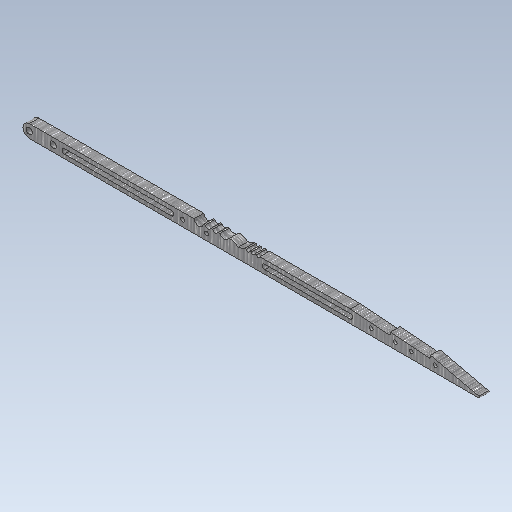
# Autodesk Inventor part: ロッド
Saved by Autodesk Inventor 2020 (Build 240168000, 168)
## iProperties
Created: 2019-12-03
Part Number: ロッド
Material: アルミニウム 7075
Document SubType Name: Modeling
Designer: tanjihayato
Density: 2.81 g/cm^3
Appearance: サテン - ブラシ仕上げ 重厚
Mass: 28.905 g
Surface Area: 93.2256 cm^2
Volume: 10.2865 cm^3
Author: tanjihayato
Autodesk Inventor part; units mm, degrees
ref_plane "YZ Plane" through (0, 0, 0) normal (1, 0, 0) x (0, 1, 0)
ref_plane "XZ Plane" through (0, 0, 0) normal (0, 1, 0) x (-1, 0, 0)
ref_plane "XY Plane" through (0, 0, 0) normal (0, 0, 1) x (1, 0, 0)
sketch "スケッチ1" plane through (0, 0, 0) normal (0, 0, 1) x (1, 0, 0)
  circle A0 centre (0, 0) radius 2
  circle A1 centre (15, 0) radius 2
  arc A2 (-0.2273, 4.9948) -> (-2.9263, -4.0542) centre (0, 0) ccw
  circle A3 centre (55, 0) radius 1.5
  circle A4 centre (55, 0) radius 4.025
  arc A5 (57.9262, 6.3865) -> (54.6807, 7.0177) centre (55, 0) ccw
  arc A6 (46.6204, -10.301) -> (48.0377, -5.2999) centre (45.4517, -7.2684) ccw
  line L0 (80, -19) -> (95, -19)
  circle A7 centre (95, -15) radius 2
  circle A8 centre (80, -15) radius 2
  arc A9 (95, -19) -> (96.6662, -11.3635) centre (95, -15) ccw
  circle A10 centre (80, -15) radius 4 construction
  line L1 (48.2385, -19) -> (80, -19)
  line L2 (57.9262, 6.3865) -> (96.6662, -11.3635)
  arc A11 (46.3293, 1.1755) -> (48.0377, -5.2999) centre (55, 0) ccw
  arc A12 (62.367, -1.4063) -> (54.6591, 7.4922) centre (55, 0) ccw
  line L3 (-0.2273, 4.9948) -> (54.6591, 7.4922)
  circle A13 centre (13, -10) radius 1.5
  arc A14 (10.3663, -13.6488) -> (12.3637, -14.4548) centre (13, -10) ccw
  line L4 (-2.9263, -4.0542) -> (10.3663, -13.6488)
  arc A15 (54.3637, -20.4538) -> (59.4202, -16.8428) centre (55, -15.999) ccw
  line L5 (12.3637, -14.4548) -> (54.3637, -20.4538)
  line L6 (59.4202, -16.8428) -> (62.367, -1.4063)
  circle A16 centre (66.7169, -2.5911) radius 1.5
  circle A17 centre (66.7169, -2.5911) radius 4.5 construction
  circle A18 centre (48.2385, -14.5) radius 1.5
  arc A19 (46.6204, -10.301) -> (48.2385, -19) centre (48.2385, -14.5) ccw
  arc A20 (80, -11) -> (80, -19) centre (80, -15) ccw
  line L7 (355.4948, -11) -> (390, -19)
  line L8 (390, -19) -> (80, -19)
  circle A21 centre (358.4948, -15) radius 1.25
  circle A22 centre (343.4948, -15) radius 1.25
  circle A23 centre (333.4948, -15) radius 1.25
  circle A24 centre (318.4948, -15) radius 1.25
  line L9 (80, -11) -> (207.8755, -11)
  line L10 (355.4948, -11) -> (248.9511, -11)
  arc A25 (213.7823, -10) -> (213.8378, -11) centre (210.8567, -10.6639) ccw
  line L11 (213.7823, -10) -> (214.7761, -9.8894)
  line L12 (213.8378, -11) -> (214.8378, -11)
  line L13 (219.357, -11) -> (218.357, -11)
  line L14 (218.2737, -9.5) -> (219.2676, -9.3894)
  line L15 (222.8762, -11) -> (223.8762, -11)
  line L16 (222.7652, -9) -> (223.7591, -8.8894)
  arc A26 (214.8378, -11) -> (218.357, -11) centre (216.5974, -10.3453) ccw
  arc A27 (218.2737, -9.5) -> (214.7761, -9.8894) centre (216.5974, -10.3453) ccw
  arc A28 (219.357, -11) -> (222.8762, -11) centre (221.1166, -10.0946) ccw
  arc A29 (222.7652, -9) -> (219.2676, -9.3894) centre (221.1166, -10.0946) ccw
  line L17 (210.8567, -10.6639) -> (233.0155, -9.4343) construction
  arc A30 (223.8762, -11) -> (229.892, -10.6107) centre (226.7628, -8.9308) ccw
  arc A31 (226.8407, -8.7739) -> (223.7591, -8.8894) centre (225.3075, -9.0352) ccw
  arc A32 (226.8407, -8.7739) -> (230.4998, -7.0068) centre (226.5478, -3.4953) ccw
  arc A33 (233.6316, -8.397) -> (230.4998, -7.0068) centre (231.2455, -9.5496) ccw
  arc A34 (235.4619, -12.6053) -> (229.892, -10.6107) centre (230.3136, -18.2076) ccw
  arc A35 (235.4619, -12.6053) -> (239.6511, -11) centre (234.0497, -2.6513) ccw
  arc A36 (259.6965, 4.4867) -> (265.8152, 14.9495) centre (248.2498, 18.2013) ccw
  arc A37 (220.191, -4.195) -> (265.8152, 14.9495) centre (219.3797, 61.6752) ccw
  line L18 (220.191, -4.195) -> (207.615, -4.3499)
  arc A38 (196.7777, -11) -> (207.615, -4.3499) centre (196.7777, 1.1554) ccw
  line L19 (222.8762, -11) -> (240.076, -10.0456) construction
  line L20 (222.7652, -9) -> (239.478, -8.0726) construction
  line L21 (239.6511, -11) -> (240.6511, -11)
  arc A39 (240.6511, -11) -> (242.7511, -11) centre (241.7011, -11) ccw
  line L22 (242.7511, -11) -> (243.7511, -11)
  arc A40 (243.7511, -11) -> (245.8511, -11) centre (244.8011, -11) ccw
  line L23 (245.8511, -11) -> (246.8511, -11)
  arc A41 (246.8511, -11) -> (248.9511, -11) centre (247.9011, -11) ccw
  arc A42 (240.735, -6.337) -> (238.7449, -7.0075) centre (239.7428, -6.6807) ccw
  arc A43 (243.5362, -5.2633) -> (241.5809, -6.0291) centre (242.5618, -5.6544) ccw
  arc A44 (246.2823, -4.0554) -> (244.3663, -4.9148) centre (245.3279, -4.4932) ccw
  arc A45 (248.9668, -2.7162) -> (247.0946, -3.6672) centre (248.0347, -3.1996) ccw
  arc A46 (233.6316, -8.397) -> (238.7449, -7.0075) centre (219.9279, 52.1342) ccw
  arc A47 (240.735, -6.337) -> (241.5809, -6.0291) centre (219.9279, 52.1342) ccw
  arc A48 (243.5362, -5.2633) -> (244.3663, -4.9148) centre (219.9279, 52.1342) ccw
  arc A49 (246.2823, -4.0554) -> (247.0946, -3.6672) centre (219.9279, 52.1342) ccw
  arc A50 (248.9668, -2.7162) -> (259.6965, 4.4867) centre (219.9279, 52.1342) ccw
  line L24 (196.7777, -11) -> (196.7777, -15)
  circle A51 centre (200.7777, -15) radius 1.25
  circle A52 centre (215.7777, -15) radius 1.25
  arc A53 (196.7777, -15) -> (200.7777, -19) centre (200.7777, -15) ccw
  arc A54 (215.7777, -19) -> (217.9536, -11.6436) centre (215.7777, -15) ccw
  circle A55 centre (200.7777, -15) radius 1.5
  circle A56 centre (215.7777, -15) radius 1.5
  line L25 (200.7777, -19) -> (215.7777, -19)
  circle A57 centre (45.4517, -7.2684) radius 1.5
  arc A58 (46.3293, 1.1755) -> (44.1782, 4.6812) centre (43.1088, 1.6121) ccw
  line L26 (54.6807, 7.0177) -> (44.8362, 6.5698)
  line L27 (44.8362, 6.5698) -> (44.1782, 4.6812)
  line L28 (355.4948, -11) -> (355.4948, -13)
  line L29 (355.4948, -13) -> (330.4948, -11)
  line L30 (330.4948, -11) -> (330.4948, -13)
  line L31 (330.4948, -13) -> (305.4948, -11)
  dimension "d0" = 4
  dimension "d1" = 4
  dimension "d2" = 15
  dimension "d3" = 3
  dimension "d4" = 3
  dimension "d8" = 8.05
  dimension "d9" = 3
  dimension "d10" = 6.5
  dimension "d11" = 4
  dimension "d12" = 4
  dimension "d15" = 15
  dimension "d16" = 15
  dimension "d18" = 3
  dimension "d19" = 3
  dimension "d23" = 3
  dimension "d25" = 40
  dimension "d26" = 40
  dimension "d28" = 15
  dimension "d29" = 13
  dimension "d34" = 3
  dimension "d35" = 3
  dimension "d36" = 3
  dimension "d37" = 8
  dimension "d38" = 390
  dimension "d40" = 4
  dimension "d41" = 8
  dimension "d42" = 2.5
  dimension "d43" = 2.5
  dimension "d44" = 2.5
  dimension "d45" = 2.5
  dimension "d46" = 4
  dimension "d47" = 15
  dimension "d48" = 10
  dimension "d49" = 15
  dimension "d51" = 6
  dimension "d59" = 1
  dimension "d60" = 1.5
  dimension "d61" = 1
  dimension "d62" = 1
  dimension "d63" = 1
  dimension "d64" = 2
  dimension "d65" = 1
  dimension "d66" = 1.0015
  dimension "d67" = 1.0015
  dimension "d68" = 0.7511
  dimension "d69" = 0.7511
  dimension "d70" = 3.176
  dimension "d71" = 3.176
  dimension "d73" = 1.05
  dimension "d74" = 1.05
  dimension "d75" = 1.05
  dimension "d76" = 1
  dimension "d77" = 1
  dimension "d78" = 1
  dimension "d79" = 2.1
  dimension "d80" = 2.1
  dimension "d81" = 2.1
  dimension "d82" = 2.1
  dimension "d83" = 3
  dimension "d84" = 3
  dimension "d85" = 3
  dimension "d88" = 2.5
  dimension "d89" = 2.5
  dimension "d90" = 15
  constraints: 91 point on circle, 64 end point, 59 centre point, 30 tangent, 15 point on line, 11 coincident, 9 horizontal, 7 collinear, 6 horizontal alignment, 3 parallel, 3 vertical, 2 concentric, 1 vertical alignment, 2 other
  measures "d0" diameter of A0
  measures "d1" diameter of A1
  measures "d2" distance of point (0, 0) A1.centre
  measures "d3" radial gap between concentric circles of A0 A2
  measures "d4" diameter of A3
  measures "d8" diameter of A4
  measures "d9" radial gap between concentric circles of A4 A5
  measures "d10" diameter of A6
  measures "d11" diameter of A7
  measures "d12" diameter of A8
  measures "d15" distance of A8.centre A7.centre
  measures "d16" diameter of A12
  measures "d18" diameter of A13
  measures "d19" radial gap between concentric circles of A13 A14
  measures "d23" diameter of A16
  measures "d25" distance of A4.centre A1.centre
  measures "d26" horizontal distance of A3.centre A7.centre
  measures "d28" vertical distance of A8.centre A3.centre
  measures "d29" horizontal distance of A13.centre point (0, 0)
  measures "d34" diameter of A18
  measures "d35" radial gap between concentric circles of A17 A16
  measures "d36" radial gap between concentric circles of A18 A19
  measures "d37" diameter of A20
  measures "d38" horizontal distance of point (0, 0) L7.end
  measures "d40" radius of A9
  measures "d41" diameter of A10
  measures "d42" diameter of A21
  measures "d43" diameter of A22
  measures "d44" diameter of A23
  measures "d45" diameter of A24
  measures "d46" distance from line of L8 A24.centre
  measures "d47" distance of A23.centre A24.centre
  measures "d48" distance of A23.centre A22.centre
  measures "d49" distance of A21.centre A22.centre
  measures "d51" diameter of A25
  measures "d59" vertical distance of L12.start L11.start
  measures "d60" vertical distance of L13.end L14.start
  measures "d61" distance of L12.start L12.end
  measures "d62" distance of L13.end L13.start
  measures "d63" distance of L15.start L15.end
  measures "d64" vertical distance of L15.start L16.start
  measures "d65" distance of L16.start L16.end
  measures "d66" distance from line of L17 L16.start
  measures "d67" distance from line of L15.start L17
  measures "d68" distance from line of L17 L14.start
  measures "d69" distance from line of L17 L13.end
  measures "d70" angle of L16 L20
  measures "d71" angle of L15 L19
  measures "d73" radius of A39
  measures "d74" radius of A40
  measures "d75" radius of A41
  measures "d76" distance of L23.start L23.end
  measures "d77" distance of L22.start L22.end
  measures "d78" distance of L21.start L21.end
  measures "d79" diameter of A42
  measures "d80" diameter of A43
  measures "d81" diameter of A44
  measures "d82" diameter of A45
  measures "d83" distance of A42.centre A43.centre
  measures "d84" distance of A44.centre A43.centre
  measures "d85" distance of A45.centre A44.centre
  measures "d88" diameter of A51
  measures "d89" diameter of A52
  measures "d90" distance of A52.centre A51.centre
extrude "押し出し1" add sketch "スケッチ1" along normal blind 6 contours L9 L24 A53 L8 A9 L2 | L2 A9 L0 A20 L9 | L9 A25 L12 A26 A54 L8 A53 L24 | A54 A26 L13 A28 L15 A30 A34 A35 L21 A39 L22 A40 L23 A41 L10 L31 L30 L29 L28 L7 L8 | A55 | A56
sketch "スケッチ2" plane through (0, 0, 6) normal (0, 0, 1) x (1, 0, 0)
  circle A0 centre (215.7777, -15) radius 1.25 projected
  circle A1 centre (200.7777, -15) radius 1.25 projected
  circle A2 centre (80, -15) radius 2 projected
  circle A3 centre (95, -15) radius 2 projected
  circle A4 centre (318.4948, -15) radius 1.25 projected
  circle A5 centre (333.4948, -15) radius 1.25 projected
  circle A6 centre (343.4948, -15) radius 1.25 projected
  circle A7 centre (358.4948, -15) radius 1.25 projected
  arc A8 (80, -11) -> (80, -19) centre (80, -15) ccw projected
  line L0 (80, -19) -> (390, -19) projected
  line L1 (390, -19) -> (355.4948, -11) projected
  line L2 (305.4948, -11) -> (248.9511, -11) projected
  arc A9 (246.8511, -11) -> (248.9511, -11) centre (247.9011, -11) ccw projected
  line L3 (246.8511, -11) -> (245.8511, -11) projected
  arc A10 (243.7511, -11) -> (245.8511, -11) centre (244.8011, -11) ccw projected
  line L4 (243.7511, -11) -> (242.7511, -11) projected
  arc A11 (240.6511, -11) -> (242.7511, -11) centre (241.7011, -11) ccw projected
  line L5 (240.6511, -11) -> (239.6511, -11) projected
  arc A12 (235.4619, -12.6053) -> (239.6511, -11) centre (234.0497, -2.6513) ccw projected
  arc A13 (235.4619, -12.6053) -> (229.892, -10.6107) centre (230.3136, -18.2076) ccw projected
  arc A14 (223.8762, -11) -> (229.892, -10.6107) centre (226.7628, -8.9308) ccw projected
  line L6 (223.8762, -11) -> (222.8762, -11) projected
  arc A15 (219.357, -11) -> (222.8762, -11) centre (221.1166, -10.0946) ccw projected
  line L7 (219.357, -11) -> (218.357, -11) projected
  arc A16 (214.8378, -11) -> (218.357, -11) centre (216.5974, -10.3453) ccw projected
  line L8 (214.8378, -11) -> (213.8378, -11) projected
  arc A17 (207.8755, -11) -> (213.8378, -11) centre (210.8567, -10.6639) ccw projected
  line L9 (207.8755, -11) -> (80, -11) projected
  circle A18 centre (105, -15) radius 2
  circle A19 centre (120, -15) radius 2
  arc A20 (105, -11) -> (105, -19) centre (105, -15) ccw
  line L10 (207.8755, -11) -> (80, -11) projected
  line L11 (330.4948, -11) -> (330.4948, -13) projected
  line L12 (330.4948, -13) -> (305.4948, -11) projected
  line L13 (355.4948, -11) -> (355.4948, -13) projected
  line L14 (355.4948, -13) -> (330.4948, -11) projected
  point P0 (0, 0)
  dimension "d114" = 4
  dimension "d115" = 4
  dimension "d116" = 15
  dimension "d117" = 4
  dimension "d119" = 25
  constraints: 3 centre point, 2 point on circle, 2 point on line, 1 coincident, 1 horizontal alignment, 1 tangent
  measures "d114" diameter of A18
  measures "d115" diameter of A19
  measures "d116" distance of A18.centre A19.centre
  measures "d117" distance from line of L9 A19.centre
  measures "d119" distance of A2.centre A18.centre
extrude "押し出し2" cut sketch "スケッチ2" against normal blind 10 contours L9 A20 L0 A8 | A18 | A19
fillet "フィレット1" radius 0.5 1 edges at (390, -19, 3)
fillet "フィレット2" radius 1 2 edges at (355.4948, -13, 3) (330.4948, -13, 3)
sketch "スケッチ3" plane through (0, 0, 6) normal (0, 0, 1) x (1, 0, 0)
  arc A0 (385.6296, -19) -> (385.7426, -18.0129) centre (385.6296, -18.5) ccw projected
  line L0 (385.7426, -18.0129) -> (355.4948, -11) projected
  line L1 (355.4948, -11) -> (355.4948, -11.9168) projected
  arc A1 (354.4151, -12.9136) -> (355.4948, -11.9168) centre (354.4948, -11.9168) ccw projected
  line L2 (354.4151, -12.9136) -> (330.4948, -11) projected
  line L3 (330.4948, -11) -> (330.4948, -11.9168) projected
  arc A2 (329.4151, -12.9136) -> (330.4948, -11.9168) centre (329.4948, -11.9168) ccw projected
  line L4 (329.4151, -12.9136) -> (305.4948, -11) projected
  line L5 (305.4948, -11) -> (248.9511, -11) projected
  arc A3 (246.8511, -11) -> (248.9511, -11) centre (247.9011, -11) ccw projected
  line L6 (246.8511, -11) -> (245.8511, -11) projected
  arc A4 (243.7511, -11) -> (245.8511, -11) centre (244.8011, -11) ccw projected
  line L7 (243.7511, -11) -> (242.7511, -11) projected
  arc A5 (240.6511, -11) -> (242.7511, -11) centre (241.7011, -11) ccw projected
  line L8 (240.6511, -11) -> (239.6511, -11) projected
  arc A6 (235.4619, -12.6053) -> (239.6511, -11) centre (234.0497, -2.6513) ccw projected
  arc A7 (235.4619, -12.6053) -> (229.892, -10.6107) centre (230.3136, -18.2076) ccw projected
  arc A8 (223.8762, -11) -> (229.892, -10.6107) centre (226.7628, -8.9308) ccw projected
  line L9 (223.8762, -11) -> (222.8762, -11) projected
  arc A9 (219.357, -11) -> (222.8762, -11) centre (221.1166, -10.0946) ccw projected
  line L10 (219.357, -11) -> (218.357, -11) projected
  arc A10 (214.8378, -11) -> (218.357, -11) centre (216.5974, -10.3453) ccw projected
  line L11 (214.8378, -11) -> (213.8378, -11) projected
  arc A11 (207.8755, -11) -> (213.8378, -11) centre (210.8567, -10.6639) ccw projected
  line L12 (207.8755, -11) -> (105, -11) projected
  arc A12 (105, -11) -> (105, -19) centre (105, -15) ccw projected
  line L13 (105, -19) -> (385.6296, -19) projected
  circle A13 centre (318.4948, -15) radius 1.25 projected
  circle A14 centre (333.4948, -15) radius 1.25 projected
  circle A15 centre (343.4948, -15) radius 1.25 projected
  circle A16 centre (358.4948, -15) radius 1.25 projected
  circle A17 centre (200.7777, -15) radius 1.25 projected
  circle A18 centre (215.7777, -15) radius 1.25 projected
  circle A19 centre (120, -15) radius 2 projected
  circle A20 centre (105, -15) radius 2 projected
  line L14 (127, -15) -> (193.7777, -15) construction
  line L15 (127, -16.5) -> (193.7777, -16.5)
  line L16 (193.7777, -13.5) -> (127, -13.5)
  arc A21 (127, -13.5) -> (127, -16.5) centre (127, -15) ccw
  arc A22 (193.7777, -16.5) -> (193.7777, -13.5) centre (193.7777, -15) ccw
  line L17 (251.9511, -15) -> (305.4948, -15) construction
  line L18 (251.9511, -16.5) -> (305.4948, -16.5)
  line L19 (305.4948, -13.5) -> (251.9511, -13.5)
  arc A23 (251.9511, -13.5) -> (251.9511, -16.5) centre (251.9511, -15) ccw
  arc A24 (305.4948, -16.5) -> (305.4948, -13.5) centre (305.4948, -15) ccw
  point P0 (0, 0)
  point P1 (160.3889, -15)
  point P2 (278.723, -15)
  dimension "d129" = 3
  dimension "d130" = 3
  dimension "d131" = 7
  dimension "d132" = 7
  dimension "d133" = 3
  dimension "d134" = 0
  constraints: 16 end point, 8 point on circle, 8 tangent, 4 centre point, 3 point on line, 2 midpoint, 2 parallel, 1 horizontal
  measures "d129" diameter of A22
  measures "d130" diameter of A24
  measures "d131" distance of A19.centre L14.start
  measures "d132" distance of A17.centre L14.end
  measures "d133" horizontal distance of L17.start L5.end
  measures "d134" horizontal distance of L17.end L4.end
extrude "押し出し3" cut sketch "スケッチ3" against normal blind 5 contours A21 L16 A22 L15 | A23 L19 A24 L18
